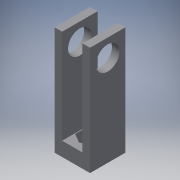
# Autodesk Inventor part: silider shaft
Saved by Autodesk Inventor 2016 (Build 200138000, 138)
## iProperties
Created: 2016-01-17
Part Number: silider shaft
Material: ABS Plastic
Document SubType Name: Modeling
Designer: gus
Density: 1.06 g/cm^3
Appearance: Smooth - Red
Author: gus
Autodesk Inventor part; units mm, degrees
ref_plane "YZ Plane" through (0, 0, 0) normal (1, 0, 0) x (0, 1, 0)
ref_plane "XZ Plane" through (0, 0, 0) normal (0, 1, 0) x (-1, 0, 0)
ref_plane "XY Plane" through (0, 0, 0) normal (0, 0, 1) x (1, 0, 0)
sketch "Sketch1" plane through (0, 0, 0) normal (0, 1, 0) x (-1, 0, 0)
  line L0 (0, 0) -> (19.05, 0)
  line L1 (19.05, 0) -> (19.05, -19.05)
  line L2 (19.05, -19.05) -> (0, -19.05)
  line L3 (0, -19.05) -> (0, 0)
  dimension "d0" = 19.05
  dimension "d1" = 19.05
  constraints: 8 end point, 2 parallel, 1 horizontal, 1 perpendicular
  measures "d0" distance between parallel lines of L3 L1
  measures "d1" distance between parallel lines of L2 L0
extrude "Extrusion1" add sketch "Sketch1" along normal blind 7.62
sketch "Sketch2" plane through (0, 7.62, 0) normal (0, 1, 0) x (1, 0, 0)
  line L0 (-9.525, 3.6591) -> (-14.605, 6.5921)
  line L1 (-14.605, 6.5921) -> (-14.605, 12.4579)
  line L2 (-14.605, 12.4579) -> (-9.525, 15.3909)
  line L3 (-9.525, 15.3909) -> (-4.445, 12.4579)
  line L4 (-4.445, 12.4579) -> (-4.445, 6.5921)
  line L5 (-4.445, 6.5921) -> (-9.525, 3.6591)
  line L6 (0, 19.05) -> (-19.05, 19.05) projected
  line L7 (0, 0) -> (0, 19.05) projected
  point P0 (-9.525, 9.525)
  dimension "d4" = 10.16
  dimension "d5" = 9.525
  dimension "d6" = 9.525
  constraints: 12 end point, 1 vertical, 13 other
  measures "d4" distance between parallel lines of L4 L1
  measures "d5" distance from line of L6 point (-9.525, 9.525)
  measures "d6" distance from line of L7 point (-9.525, 9.525)
extrude "Extrusion2" cut sketch "Sketch2" against normal blind 6.35
sketch "Sketch3" plane through (0, 1.27, 0) normal (0, 1, 0) x (1, 0, 0)
  circle A0 centre (-9.525, 9.525) radius 2.413
  line L0 (-14.605, 12.4579) -> (-9.525, 15.3909) projected
  line L1 (-9.525, 3.6591) -> (-14.605, 6.5921) projected
  point P0 (0, 0)
  dimension "d9" = 4.826
  dimension "d10" = 5.08
  dimension "d11" = 5.08
  constraints: 1 centre point
  measures "d9" diameter of A0
  measures "d10" distance from line of L0 A0.centre
  measures "d11" distance from line of L1 A0.centre
extrude "Extrusion3" cut sketch "Sketch3" against normal blind 12.7
sketch "Sketch4" plane through (0, 7.62, 0) normal (0, 1, 0) x (1, 0, 0)
  line L0 (0, 19.05) -> (-19.05, 19.05) projected
  line L1 (-19.05, 19.05) -> (-14.986, 19.05)
  line L2 (-14.986, 19.05) -> (-14.986, 0)
  line L3 (-14.986, 0) -> (-19.05, 0)
  line L4 (-19.05, 0) -> (-19.05, 19.05)
  line L5 (0, 19.05) -> (-4.064, 19.05)
  line L6 (-4.064, 19.05) -> (-4.064, 0)
  line L7 (-4.064, 0) -> (0, 0)
  line L8 (0, 0) -> (0, 19.05)
  line L9 (-19.05, 0) -> (0, 0) projected
  dimension "d14" = 4.064
  dimension "d15" = 4.064
  constraints: 16 end point, 4 parallel, 2 collinear, 2 horizontal, 2 perpendicular
  measures "d14" distance between parallel lines of L4 L2
  measures "d15" distance between parallel lines of L6 L8
extrude "Extrusion4" add sketch "Sketch4" along normal blind 50.8 contours L8 L7 L6 L0 | L2 L3 L4 L0
sketch "Sketch5" plane through (-19.05, 0, -19.05) normal (-1, 0, 0) x (0, 0, 1)
  circle A0 centre (9.525, 48.895) radius 6.35
  line L0 (19.05, 0) -> (19.05, 58.42) projected
  line L1 (0, 58.42) -> (19.05, 58.42) projected
  dimension "d18" = 12.7
  dimension "d19" = 9.525
  dimension "d20" = 9.525
  constraints: 1 centre point
  measures "d18" diameter of A0
  measures "d19" distance from line of L0 A0.centre
  measures "d20" distance from line of L1 A0.centre
extrude "Extrusion5" cut sketch "Sketch5" against normal blind 19.05
body "Solid1"
